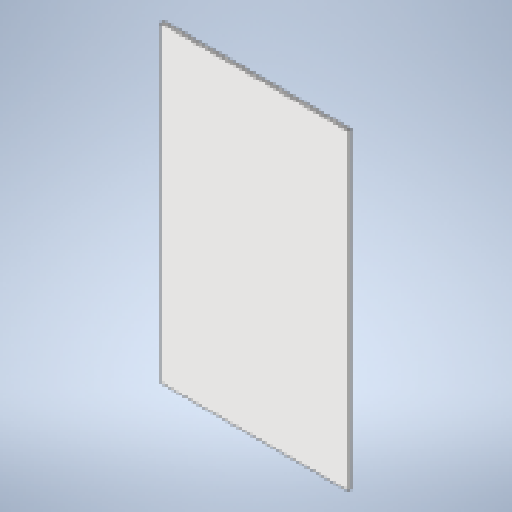
# Autodesk Inventor part: SLM- Floordummy
Saved by Autodesk Inventor 2025.4 (Build 294407000, 407)
## iProperties
Created: 2026-02-19
Part Number: SLM- Floordummy
Material: Generic
Document SubType Name: Modeling
Designer: admin
Density: 1 g/cm^3
Appearance: Default
Author: admin
Autodesk Inventor part; units mm, degrees
ref_plane "YZ Plane" through (0, 0, 0) normal (1, 0, 0) x (0, 1, 0)
ref_plane "XZ Plane" through (0, 0, 0) normal (0, 1, 0) x (-1, 0, 0)
ref_plane "XY Plane" through (0, 0, 0) normal (0, 0, 1) x (1, 0, 0)
sketch "Sketch1" plane through (0, 0, 0) normal (0, 0, 1) x (1, 0, 0)
  line L0 (2400, -4000) -> (-2400, -4000)
  line L1 (-2400, -4000) -> (-2400, 4000)
  line L2 (-2400, 4000) -> (2400, 4000)
  line L3 (2400, 4000) -> (2400, -4000)
  line L4 (2400, -4000) -> (-2400, 4000) construction
  line L5 (-2400, -4000) -> (2400, 4000) construction
  point P0 (0, 0)
  dimension "d0" = 4800
  dimension "d1" = 8000
  constraints: 12 end point, 2 midpoint, 2 parallel, 1 horizontal, 1 perpendicular
  measures "d0" distance of L1.end L2.end
  measures "d1" distance of L0.end L1.end
extrude "Extrusion1" add sketch "Sketch1" along normal blind 80
body "Solid1"
